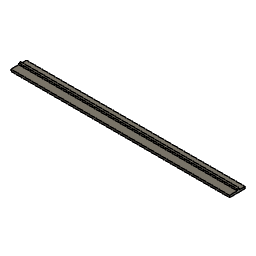
guiderail (Autodesk Fusion 360 design; units mm, degrees)
Autodesk Fusion 360 part; units mm, degrees
sketch "Sketch1" plane through (0, 0, 0) normal (0, 1, 0) x (1, 0, 0)
  line L0 (0, 0) -> (170, 0)
  line L1 (170, 0) -> (170, -12)
  line L2 (170, -12) -> (0, -12)
  line L3 (0, -12) -> (0, 0)
  dimension "d1" = 170
  dimension "d2" = 12
  constraint horizontal L0
  constraint vertical L1
  constraint horizontal L2
  constraint vertical L3
  constraint coincident L0.start L3.end
  measures "d1" distance of L0.start L0.end
  measures "d2" distance of L0.start L2.end
extrude "Extrude1" add sketch "Sketch1" along normal blind 1.5
sketch "Sketch2" plane through (0, 1.5, 0) normal (0, 1, 0) x (-1, 0, 0)
  line L0 (0, 12) -> (-170, 12)
  line L1 (-170, 12) -> (-170, 0)
  line L2 (-170, 0) -> (0, 0)
  line L3 (0, 0) -> (0, 12)
  line L4 (-170, 6) -> (0, 6)
  line L5 (0, 6) -> (0, 4.5)
  line L6 (0, 4.5) -> (-170, 4.5)
  line L7 (-170, 4.5) -> (-170, 6)
  dimension "d5" = 1.5
  constraint horizontal L4
  constraint vertical L5
  constraint horizontal L6
  constraint vertical L7
  constraint coincident L3 L5.end
  constraint midpoint L1 L4.start
  measures "d5" distance of L4 L6
extrude "Extrude2" add sketch "Sketch2" along normal blind 1.25 contours L1 L3 L4 L5 L6 L7
equation "d1 = 125 mm + 40 mm + 5 mm"
